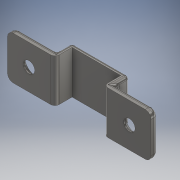
# Autodesk Inventor part: Latch Catch
Saved by Autodesk Inventor 2018 (Build 220112000, 112)
## iProperties
Created: 2018-10-16
Part Number: Latch Catch
Material: Steel
Document SubType Name: Modeling
Designer: P301319
Density: 7.85 g/cm^3
Appearance: Semi-Polished
Author: P301319
Autodesk Inventor part; units mm, degrees
ref_plane "YZ Plane" through (0, 0, 0) normal (1, 0, 0) x (0, 1, 0)
ref_plane "XZ Plane" through (0, 0, 0) normal (0, 1, 0) x (-1, 0, 0)
ref_plane "XY Plane" through (0, 0, 0) normal (0, 0, 1) x (1, 0, 0)
sketch "Sketch1" plane through (0, 0, 0) normal (0, 0, 1) x (1, 0, 0)
  line L0 (0, 0) -> (50, 0) construction
  line L1 (0, 0) -> (16.5, 0)
  line L2 (50, 0) -> (33.5, 0)
  line L3 (0, 0) -> (0, 2.5)
  line L4 (50, 0) -> (50, 2.5)
  line L5 (16.5, 0) -> (16.5, 6)
  line L6 (33.5, 0) -> (33.5, 6)
  line L7 (33.5, 6) -> (16.5, 6)
  line L8 (0, 2.5) -> (15, 2.5)
  line L9 (50, 2.5) -> (35, 2.5)
  line L10 (15, 2.5) -> (15, 7.5)
  line L11 (35, 2.5) -> (35, 7.5)
  line L12 (15, 7.5) -> (35, 7.5)
  dimension "d0" = 50
  dimension "d1" = 16.5
  dimension "d2" = 16.5
  dimension "d3" = 2.5
  dimension "d4" = 6
  dimension "d5" = 15
  dimension "d6" = 15
  dimension "d7" = 2.5
  dimension "d8" = 5
  dimension "d9" = 5
  constraints: 26 end point, 5 vertical, 4 horizontal, 2 point on line, 1 perpendicular
  measures "d0" distance of L0.start L0.end
  measures "d1" distance of L0.start L1.end
  measures "d2" distance of L0.end L2.end
  measures "d3" distance of L0.start L3.end
  measures "d4" distance of L1.end L5.end
  measures "d5" distance of L3.end L8.end
  measures "d6" distance of L4.end L9.end
  measures "d7" distance of L0.end L4.end
  measures "d8" distance of L8.end L10.end
  measures "d9" distance of L9.end L11.end
extrude "Extrusion1" add sketch "Sketch1" along normal blind 15
sketch "Sketch2" plane through (35, 2.5, 0) normal (0, 1, 0) x (1, 0, 0)
  line L0 (15, 0) -> (15, -15) projected
  line L1 (-35, 0) -> (-35, -15) projected
  point P0 (7.5, -7.5)
  point P1 (-27.5, -7.5)
  point P2 (15, -7.5)
  dimension "d12" = 7.5
  dimension "d13" = 7.5
  constraints: 2 horizontal alignment, 1 midpoint
  measures "d12" distance from line of L0 point (7.5, -7.5)
  measures "d13" distance from line of L1 point (-27.5, -7.5)
hole "Hole1" at (42.5, 2.5, 7.5) at (7.5, 2.5, 7.5) direction (0, -1, 0) diameter 4 end through all countersink diameter 8 countersink angle 90
fillet "Fillet1" radius 1 10 edges at (7.5, 2.5, 3.5) (42.5, 2.5, 3.5) (25, 7.5, 15) (35, 5, 15) (15, 5, 15) (15, 5, 0) (25, 7.5, 0) (35, 5, 0) (35, 7.5, 7.5) (15, 7.5, 7.5)
fillet "Fillet2" radius 1.5 12 edges at (34.5, 2.5, 15) (42.5, 2.5, 15) (50, 2.5, 7.5) (34.5, 2.5, 0) (42.5, 2.5, 0) (15.5, 2.5, 0) (7.5, 2.5, 0) (0, 2.5, 7.5) (15.5, 2.5, 15) (7.5, 2.5, 15) (16.5, 0, 7.5) (33.5, 0, 7.5)
fillet "Fillet3" radius 2 8 edges at (49.5607, 2.0607, 14.5607) (50, 0.5, 15) (50, 0.5, 0) (49.5607, 2.0607, 0.4393) (0, 0.5, 15) (0.4393, 2.0607, 14.5607) (0, 0.5, 0) (0.4393, 2.0607, 0.4393)
fillet "Fillet4" radius 1.5 10 edges at (35, 2.4784, 13.7537) (34.6379, 1.798, 14.7701) (35, 2.4784, 1.2463) (34.6379, 1.798, 0.2299) (35, 2.5, 7.5) (15, 2.4784, 13.7537) (15, 2.5, 7.5) (15, 2.4784, 1.2463) (15.3621, 1.798, 0.2299) (15.3621, 1.798, 14.7701)
equation "\"d2\" = d1"
equation "\"d6\" = d5"
equation "\"d7\" = d3"
equation "\"d9\" = d8"
equation "\"d13\" = d12"
body "Solid1"
